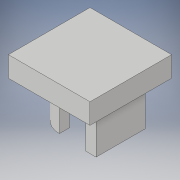
# Autodesk Inventor part: 2
Saved by Autodesk Inventor 2019 (Build 230136000, 136)
## iProperties
Created: 2018-08-09
Part Number: 2
Material: Generic
Document SubType Name: Modeling
Designer: Ge Shi
Density: 1 g/cm^3
Appearance: Default
Author: Ge Shi
Autodesk Inventor part; units mm, degrees
ref_plane "YZ Plane" through (0, 0, 0) normal (1, 0, 0) x (0, 1, 0)
ref_plane "XZ Plane" through (0, 0, 0) normal (0, 1, 0) x (-1, 0, 0)
ref_plane "XY Plane" through (0, 0, 0) normal (0, 0, 1) x (1, 0, 0)
sketch "Sketch1" plane through (0, 0, 0) normal (0, 1, 0) x (-1, 0, 0)
  line L0 (-10, -10) -> (10, -10)
  line L1 (10, -10) -> (10, 10)
  line L2 (10, 10) -> (-10, 10)
  line L3 (-10, 10) -> (-10, -10)
  line L4 (-10, -10) -> (10, 10) construction
  line L5 (10, -10) -> (-10, 10) construction
  point P0 (0, 0)
  dimension "d0" = 20
  dimension "d1" = 20
  constraints: 12 end point, 2 midpoint, 2 parallel, 1 horizontal, 1 perpendicular
  measures "d0" distance of L2.end L1.end
  measures "d1" distance of L0.end L1.end
extrude "Extrusion1" add sketch "Sketch1" along normal blind 5
sketch "Sketch2" plane through (0, 0, 0) normal (0, 1, 0) x (-1, 0, 0)
  arc A0 (-2.7434, -2.7839) -> (2, 5.5) centre (2, 0) ccw
  line L0 (2, 0) -> (-2.7434, -2.7839) construction
  line L1 (2, 0) -> (2, 5.5) construction
  arc A1 (-0.5873, -1.5185) -> (2, 3) centre (2, 0) ccw
  line L2 (2, 5.5) -> (2, 3)
  line L3 (-0.5873, -1.5185) -> (-5, 6)
  line L4 (-5, 6) -> (-7.5, 6)
  line L5 (-7.5, 6) -> (-7.5, -6)
  line L6 (-7.5, -6) -> (-5, -6)
  line L7 (-5, -6) -> (-5, 1.061)
  line L8 (-5, 1.061) -> (-2.7434, -2.7839)
  line L9 (-10, 10) -> (-10, -10) projected
  line L10 (7.5, 0) -> (7.5, -3.2169) construction
  line L11 (10, -10) -> (10, 10) projected
  line L12 (14, 0) -> (-14, 0) projected
  point P0 (0, 0)
  point P1 (2, 4.25)
  point P2 (-5, -2.4695)
  point P3 (-7.5, 0)
  dimension "d6" = 2.5
  dimension "d7" = 2.5
  dimension "d9" = 3
  dimension "d11" = 12
  dimension "d13" = 2.5
  dimension "d14" = 2.5
  dimension "d15" = 2.5
  constraints: 20 end point, 5 point on circle, 4 perpendicular, 3 midpoint, 2 centre point, 2 point on line, 2 tangent, 1 coincident, 1 collinear, 1 parallel, 1 vertical, 1 other
  measures "d6" distance of L5.end L6.end
  measures "d7" distance between parallel lines of L3 L8
  measures "d9" radius of A1
  measures "d11" distance of L4.end L5.end
  measures "d13" distance between parallel lines of L9 L5
  measures "d14" distance between parallel lines of L11 L10
  measures "d15" distance of L3.end L4.end
extrude "Extrusion2" add sketch "Sketch2" against normal blind 10 contours L8 L12 L3 A1 A0 | L12 A1 L2 A0 | L8 L7 L12 L5 L4 L3 | L7 L6 L5 L12
body "Solid1"
